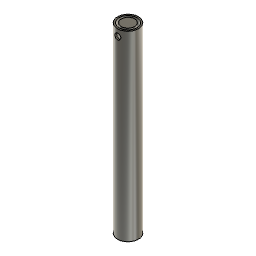
Computer Monitor Riser HUANO legs extension. Taller v16 (Autodesk Fusion 360 design; units mm, degrees)
Autodesk Fusion 360 part; units mm, degrees
note: some values were not read from the file. Chosen so that the rebuilt part matches the saved one: which bodies a step acts on; which face or edge a step refers to.
sketch "Sketch1" plane through (0, 0, 0) normal (0, 0, 1) x (1, 0, 0)
  circle A0 centre (0, 0) radius 11.25
  circle A1 centre (0, 0) radius 13.25
  dimension "d1" = 22.5
  dimension "d2" = 2
  constraint coincident A0.centre A1.centre
  measures "d1" diameter of A0
extrude "Extrude1" add sketch "Sketch1" against normal blind 171.45 contours A0 | A1 makes body 1
extrude "Extrude2" add sketch "Sketch1" along normal blind 10 bodies 1
extrude "Extrude3" add 1 faces at (12.4921, -1.2172, 10) along direction (0, 0, 1) blind 10 on bodies 1 bodies 1
sketch "Sketch2" plane through (0, 0, -171.45) normal (0, 0, -1) x (1, 0, 0)
  circle A0 centre (0, 0) radius 13.25
  circle A1 centre (0, 0) radius 13.25
  circle A2 centre (0, 0) radius 9.5
  dimension "d9" = -3.75
extrude "Extrude4" cut sketch "Sketch2" against normal blind 40 draft -1 contours A2 bodies 1
extrude "Extrude5" add 1 faces at (12.4921, -1.2172, 20) along direction (0, 0, 1) blind 20 on bodies 1 bodies 1
sketch "Sketch3" plane through (0, 0, 0) normal (0, 0, 1) x (-1, 0, 0)
  circle A0 centre (0, 0) radius 11.25
  circle A1 centre (0, 0) radius 8.5
  dimension "d14" = 17
  constraint coincident A0.centre A1.centre
  measures "d14" diameter of A1
extrude "Extrude6" add sketch "Sketch3" along normal blind 11.5 contours A1 bodies 1
sketch "Sketch4" plane through (0, 0, 11.5) normal (0, 0, 1) x (-1, 0, 0)
  circle A0 centre (0, 0) radius 8.5
  line L0 (0, 0) -> (8.5, 0)
  line L1 (0, 0) -> (0, -8.5)
  line L2 (0, 0, 0) -> (0, 0, 5)
  dimension "d17" = 5
  constraint coincident A0.centre L0.start
  constraint coincident A0 L0.end
  constraint horizontal L0
  constraint coincident A0 L1.end
  constraint perpendicular L0 L1
  measures "d17" distance of A0.centre L0.start
ref_plane "WorkPlane1" through (0, 0, 11.5) normal (0, -1, 0) x (1, 0, 0)
split "Split1" by plane through (0, 0, 11.5) normal (0, 0, 1) bodies 1 makes body 2 at (13.1842, 1.3193, 21)
sketch "Sketch5" plane through (0, 0, 0) normal (0, -1, 0) x (-1, 0, 0)
  circle A0 centre (0, -11.5) radius 1.3
  circle A1 centre (0, -11.5) radius 3.75
  line L0 (0, -11.5) -> (0, -10.2)
  line L1 (0, -10.2) -> (0, -14.3)
  circle A2 centre (0, -11.5) radius 2.8
  line L2 (0, -14.3) -> (2.4249, -12.9)
  line L3 (2.4249, -12.9) -> (2.4249, -10.1)
  line L4 (2.4249, -10.1) -> (0, -8.7)
  line L5 (0, -8.7) -> (-2.4249, -10.1)
  line L6 (-2.4249, -10.1) -> (-2.4249, -12.9)
  line L7 (-2.4249, -12.9) -> (0, -14.3)
  point P0 (0, -11.5)
  point P1 (0, -11.5)
  dimension "d18" = 2.6
  dimension "d19" = 7.5
  dimension "d32" = 4.1
  constraint coincident P0 A0.centre
  constraint coincident P1 P0
  constraint coincident A0 L0.end
  constraint vertical L0
  constraint parallel L0 L1
  constraint coincident L1.end A2
  constraint coincident L1.end L2.start
  measures "d18" diameter of A0
  measures "d19" diameter of A1
  measures "d32" distance of L0.end L1.end
extrude "Extrude7" add sketch "Sketch4" along normal blind 28.5 bodies 1
extrude "Extrude8" cut sketch "Sketch5" along normal blind 10 contours A0 L0 L1 | A0 L0 L1 bodies 1
split "Split2" by plane through (0, 0, 0) normal (0, 0, 1) bodies 1 makes body 3 at (13.2335, 0.6605, 3.8333) makes body 4 at (2.5157, -8.1192, 17.149)
extrude "Extrude9" cut sketch "Sketch5" along normal blind 27 contours A0 L0 L1 | A0 L0 L1 | A1 | A2 L3 | A2 L4 | L2 L3 L4 L5 L6 L7 | A2 L2 | A2 L5 | A2 L7 | A2 L6 bodies 2 3
combine "Combine1" operation add target body 4 tool bodies 2 3 1
split "Split3" by plane through (0, 0, 0) normal (0, 0, 1) bodies 4 makes body 5 at (13.1842, 1.3193, 13.3333) makes body 6 at (2.5157, -8.1192, 17.149)
move_body "Move1" bodies 6 5 to x (1, 0, 0) y (0, 1, 0) z (0, 0, 1) at (0, 0, 20)
extrude "Extrude10" add 3 faces at (10.2598, -0.9812, 0) (12.534, 0.6583, 0) (2.5527, -1.2293, 0) along direction (0, 0, 1) blind 20 on bodies 4 bodies 4 5 6
extrude "Extrude11" cut 2 faces at (12.4921, -1.2172, 60) (-1.6723, -2.628, 60) along direction (0, 0, -1) blind 20 on bodies 4 bodies 4
split "Split4" by plane through (0, 0, 20) normal (0, 0, 1) bodies 4 makes body 7 at (-5.7001, -11.9612, 30.5) makes body 8 at (2.5158, -8.1192, 30.4833)
move_body "Move2" bodies 8 7 to x (1, 0, 0) y (0, 1, 0) z (0, 0, 1) at (0, 0, 20)
extrude "Extrude12" add 2 faces at (2.5527, -1.2293, 40) (12.534, 0.6583, 40) along direction (0, 0, -1) blind 20 on bodies 7 8 bodies 4 8 7
extrude "Extrude13" add sketch "Sketch5" along normal blind 5 separate body contours A2 L3 | A2 L4 | L2 L3 L4 L5 L6 L7 | A2 L2 | A2 L5 | A2 L7 | A2 L6 makes body 9
move_body "Move3" bodies 9 to x (1, 0, 0) y (0, 1, 0) z (0, 0, 1) at (0, -8.5013, 40)
extrude "Extrude14" add 1 faces at (1.773, -13.5013, 50.0447) along direction (0, -1, 0) blind 2 on bodies 9 bodies 9
move_body "Move4" bodies 9 to x (1, 0, 0) y (0, 1, 0) z (0, 0, 1) at (0, 2, 0)
extrude "Extrude15" cut 1 faces at (-1.6723, -2.628, 60) along direction (0, 0, -1) blind 15 on bodies 4 bodies 9
extrude "Extrude16" add sketch "Sketch5" along normal blind 5 separate body contours L2 L3 L4 L5 L6 L7 makes body 10
move_body "Move5" bodies 10 to x (1, 0, 0) y (0, 1, 0) z (0, 0, 1) at (0, -8.5013, 40)
extrude "Extrude17" add 1 faces at (0.9963, -8.5013, 53.2904) along direction (0, 1, 0) blind 2 on bodies 10 bodies 10
extrude "Extrude18" cut 1 faces at (-1.6723, -2.628, 60) along direction (0, 0, -1) blind 15 on bodies 4 bodies 10
hidden bodies 9 10
equation "d9 = -6.5 mm / 2 - 0.5 mm"
